Autodesk Inventor part; units mm, degrees
(part 2 of 2)
  arc A592 (44.2126, 82.716) -> (44.7772, 86.4762) centre (21.6675, 88.0234) ccw
  arc A593 (45.2915, 82.1302) -> (44.2126, 82.716) centre (0, 0) ccw
  arc A594 (48.1377, 84.6516) -> (45.2915, 82.1302) centre (62.0216, 66.1129) ccw
  arc A595 (49.2416, 84.0143) -> (48.1377, 84.6516) centre (0, 0) ccw
  arc A596 (48.481, 80.2887) -> (49.2416, 84.0143) centre (26.2446, 86.7687) ccw
  arc A597 (49.5278, 79.6472) -> (48.481, 80.2887) centre (0, 0) ccw
  arc A598 (52.502, 82.0163) -> (49.5278, 79.6472) centre (65.3967, 62.7763) ccw
  arc A599 (53.5711, 81.322) -> (52.502, 82.0163) centre (0, 0) ccw
  arc A600 (52.6166, 77.6414) -> (53.5711, 81.322) centre (30.7498, 85.2763) ccw
  arc A601 (53.6284, 76.946) -> (52.6166, 77.6414) centre (0, 0) ccw
  arc A602 (56.7225, 79.1561) -> (53.6284, 76.946) centre (68.5925, 59.2677) ccw
  arc A603 (57.7538, 78.4069) -> (56.7225, 79.1561) centre (0, 0) ccw
  arc A604 (56.6079, 74.7812) -> (57.7538, 78.4069) centre (35.1706, 83.5501) ccw
  arc A605 (57.5819, 74.0339) -> (56.6079, 74.7812) centre (0, 0) ccw
  arc A606 (60.7875, 76.079) -> (57.5819, 74.0339) centre (71.6004, 55.5966) ccw
  arc A607 (61.7781, 75.2768) -> (60.7875, 76.079) centre (0, 0) ccw
  arc A608 (60.4441, 71.7161) -> (61.7781, 75.2768) centre (39.4951, 81.5949) ccw
  arc A609 (61.3776, 70.9188) -> (60.4441, 71.7161) centre (0, 0) ccw
  arc A610 (64.6858, 72.7934) -> (61.3776, 70.9188) centre (74.4119, 51.7731) ccw
  arc A611 (65.6331, 71.9405) -> (64.6858, 72.7934) centre (0, 0) ccw
  arc A612 (64.1146, 68.4544) -> (65.6331, 71.9405) centre (43.7113, 79.4161) ccw
  arc A613 (65.0051, 67.6093) -> (64.1146, 68.4544) centre (0, 0) ccw
  arc A614 (68.4069, 69.3082) -> (65.0051, 67.6093) centre (77.0195, 47.8077) ccw
  arc A615 (69.3082, 68.4069) -> (68.4069, 69.3082) centre (0, 0) ccw
  arc A616 (67.6093, 65.0051) -> (69.3082, 68.4069) centre (47.8077, 77.0195) ccw
  arc A617 (68.4544, 64.1146) -> (67.6093, 65.0051) centre (0, 0) ccw
  arc A618 (71.9405, 65.6331) -> (68.4544, 64.1146) centre (79.4161, 43.7113) ccw
  arc A619 (72.7934, 64.6858) -> (71.9405, 65.6331) centre (0, 0) ccw
  arc A620 (70.9188, 61.3776) -> (72.7934, 64.6858) centre (51.7731, 74.4119) ccw
  arc A621 (71.7161, 60.4441) -> (70.9188, 61.3776) centre (0, 0) ccw
  arc A622 (75.2768, 61.7781) -> (71.7161, 60.4441) centre (81.5949, 39.4951) ccw
  arc A623 (76.079, 60.7875) -> (75.2768, 61.7781) centre (0, 0) ccw
  arc A624 (74.0339, 57.5819) -> (76.079, 60.7875) centre (55.5966, 71.6004) ccw
  arc A625 (74.7812, 56.6079) -> (74.0339, 57.5819) centre (0, 0) ccw
  arc A626 (78.4069, 57.7538) -> (74.7812, 56.6079) centre (83.5501, 35.1706) ccw
  arc A627 (79.1561, 56.7225) -> (78.4069, 57.7538) centre (0, 0) ccw
  arc A628 (76.946, 53.6284) -> (79.1561, 56.7225) centre (59.2677, 68.5925) ccw
  arc A629 (77.6414, 52.6166) -> (76.946, 53.6284) centre (0, 0) ccw
  arc A630 (81.322, 53.5711) -> (77.6414, 52.6166) centre (85.2763, 30.7498) ccw
  arc A631 (82.0163, 52.502) -> (81.322, 53.5711) centre (0, 0) ccw
  arc A632 (79.6472, 49.5278) -> (82.0163, 52.502) centre (62.7763, 65.3967) ccw
  arc A633 (80.2887, 48.481) -> (79.6472, 49.5278) centre (0, 0) ccw
  arc A634 (84.0143, 49.2416) -> (80.2887, 48.481) centre (86.7687, 26.2446) ccw
  arc A635 (84.6516, 48.1377) -> (84.0143, 49.2416) centre (0, 0) ccw
  arc A636 (82.1302, 45.2915) -> (84.6516, 48.1377) centre (66.1129, 62.0216) ccw
  arc A637 (82.716, 44.2126) -> (82.1302, 45.2915) centre (0, 0) ccw
  arc A638 (86.4762, 44.7772) -> (82.716, 44.2126) centre (88.0234, 21.6675) ccw
  arc A639 (87.055, 43.6414) -> (86.4762, 44.7772) centre (0, 0) ccw
  arc A640 (84.388, 40.9311) -> (87.055, 43.6414) centre (69.2682, 58.4765) ccw
  arc A641 (84.9165, 39.823) -> (84.388, 40.9311) centre (0, 0) ccw
  arc A642 (88.7012, 40.19) -> (84.9165, 39.823) centre (89.0367, 17.031) ccw
  arc A643 (89.2197, 39.0255) -> (88.7012, 40.19) centre (0, 0) ccw
  arc A644 (86.4145, 36.4585) -> (89.2197, 39.0255) centre (72.2337, 54.7712) ccw
  arc A645 (86.8843, 35.3242) -> (86.4145, 36.4585) centre (0, 0) ccw
  arc A646 (90.683, 35.4926) -> (86.8843, 35.3242) centre (89.806, 12.3479) ccw
  arc A647 (91.1398, 34.3026) -> (90.683, 35.4926) centre (0, 0) ccw
  arc A648 (88.2042, 31.8859) -> (91.1398, 34.3026) centre (75.0012, 50.9157) ccw
  arc A649 (88.614, 30.7287) -> (88.2042, 31.8859) centre (0, 0) ccw
  arc A650 (92.4163, 30.698) -> (88.614, 30.7287) centre (90.3292, 7.6309) ccw
  arc A651 (92.8102, 29.4857) -> (92.4163, 30.698) centre (0, 0) ccw
  arc A652 (89.7521, 27.226) -> (92.8102, 29.4857) centre (77.5632, 46.9207) ccw
  arc A653 (90.1008, 26.0488) -> (89.7521, 27.226) centre (0, 0) ccw
  arc A654 (93.8962, 25.8193) -> (90.1008, 26.0488) centre (90.6048, 2.8929) ccw
  arc A655 (94.2261, 24.588) -> (93.8962, 25.8193) centre (0, 0) ccw
  arc A656 (91.054, 22.4914) -> (94.2261, 24.588) centre (79.9125, 42.797) ccw
  arc A657 (91.3406, 21.2976) -> (91.054, 22.4914) centre (0, 0) ccw
  arc A658 (95.1188, 20.8697) -> (91.3406, 21.2976) centre (90.632, -1.8529) ccw
  arc A659 (95.3839, 19.6229) -> (95.1188, 20.8697) centre (0, 0) ccw
  arc A660 (92.1063, 17.6952) -> (95.3839, 19.6229) centre (82.0428, 38.5561) ccw
  arc A661 (92.33, 16.4881) -> (92.1063, 17.6952) centre (0, 0) ccw
  arc A662 (96.0807, 15.863) -> (92.33, 16.4881) centre (90.4108, -6.5937) ccw
  arc A663 (96.2801, 14.604) -> (96.0807, 15.863) centre (0, 0) ccw
  arc A664 (92.9062, 12.8505) -> (96.2801, 14.604) centre (83.9482, 34.2094) ccw
  arc A665 (93.0664, 11.6333) -> (92.9062, 12.8505) centre (0, 0) ccw
  arc A666 (96.7792, 10.8128) -> (93.0664, 11.6333) centre (89.9418, -11.3164) ccw
  arc A667 (96.9125, 9.545) -> (96.7792, 10.8128) centre (0, 0) ccw
  arc A668 (93.4514, 7.9705) -> (96.9125, 9.545) centre (85.6236, 29.769) ccw
  arc A669 (93.5477, 6.7466) -> (93.4514, 7.9705) centre (0, 0) ccw
  arc A670 (97.2125, 5.7329) -> (93.5477, 6.7466) centre (89.2263, -16.0081) ccw
  arc A671 (97.2792, 4.46) -> (97.2125, 5.7329) centre (0, 0) ccw
  arc A672 (93.7404, 3.0687) -> (97.2792, 4.46) centre (87.0642, 25.2471) ccw
  arc A673 (93.7726, 1.8415) -> (93.7404, 3.0687) centre (0, 0) ccw
  arc A674 (97.3793, 0.6374) -> (93.7726, 1.8415) centre (88.2662, -20.6559) ccw
  arc A675 (97.3793, -0.6374) -> (97.3793, 0.6374) centre (0, 0) ccw
  arc A676 (93.7726, -1.8415) -> (97.3793, -0.6374) centre (88.2662, 20.6559) ccw
  arc A677 (93.7404, -3.0687) -> (93.7726, -1.8415) centre (0, 0) ccw
  arc A678 (97.2792, -4.46) -> (93.7404, -3.0687) centre (87.0642, -25.2471) ccw
  arc A679 (97.2125, -5.7329) -> (97.2792, -4.46) centre (0, 0) ccw
  arc A680 (93.5477, -6.7466) -> (97.2125, -5.7329) centre (89.2263, 16.0081) ccw
  arc A681 (93.4514, -7.9705) -> (93.5477, -6.7466) centre (0, 0) ccw
  arc A682 (96.9125, -9.545) -> (93.4514, -7.9705) centre (85.6236, -29.769) ccw
  arc A683 (96.7792, -10.8128) -> (96.9125, -9.545) centre (0, 0) ccw
  arc A684 (93.0664, -11.6333) -> (96.7792, -10.8128) centre (89.9418, 11.3164) ccw
  arc A685 (92.9062, -12.8505) -> (93.0664, -11.6333) centre (0, 0) ccw
  arc A686 (96.2801, -14.604) -> (92.9062, -12.8505) centre (83.9482, -34.2094) ccw
  arc A687 (96.0807, -15.863) -> (96.2801, -14.604) centre (0, 0) ccw
  arc A688 (92.33, -16.4881) -> (96.0807, -15.863) centre (90.4108, 6.5937) ccw
  arc A689 (92.1063, -17.6952) -> (92.33, -16.4881) centre (0, 0) ccw
  arc A690 (95.3839, -19.6229) -> (92.1063, -17.6952) centre (82.0428, -38.5561) ccw
  arc A691 (95.1188, -20.8697) -> (95.3839, -19.6229) centre (0, 0) ccw
  arc A692 (91.3406, -21.2976) -> (95.1188, -20.8697) centre (90.632, 1.8529) ccw
  arc A693 (91.054, -22.4914) -> (91.3406, -21.2976) centre (0, 0) ccw
  arc A694 (94.2261, -24.588) -> (91.054, -22.4914) centre (79.9125, -42.797) ccw
  arc A695 (93.8962, -25.8193) -> (94.2261, -24.588) centre (0, 0) ccw
  arc A696 (90.1008, -26.0488) -> (93.8962, -25.8193) centre (90.6048, -2.8929) ccw
  arc A697 (89.7521, -27.226) -> (90.1008, -26.0488) centre (0, 0) ccw
  arc A698 (92.8102, -29.4857) -> (89.7521, -27.226) centre (77.5632, -46.9207) ccw
  arc A699 (92.4163, -30.698) -> (92.8102, -29.4857) centre (0, 0) ccw
  arc A700 (88.614, -30.7287) -> (92.4163, -30.698) centre (90.3292, -7.6309) ccw
  arc A701 (88.2042, -31.8859) -> (88.614, -30.7287) centre (0, 0) ccw
  arc A702 (91.1398, -34.3026) -> (88.2042, -31.8859) centre (75.0012, -50.9157) ccw
  arc A703 (90.683, -35.4926) -> (91.1398, -34.3026) centre (0, 0) ccw
  arc A704 (86.8843, -35.3242) -> (90.683, -35.4926) centre (89.806, -12.3479) ccw
  arc A705 (86.4145, -36.4585) -> (86.8843, -35.3242) centre (0, 0) ccw
  arc A706 (89.2197, -39.0255) -> (86.4145, -36.4585) centre (72.2337, -54.7712) ccw
  arc A707 (88.7012, -40.19) -> (89.2197, -39.0255) centre (0, 0) ccw
  arc A708 (84.9165, -39.823) -> (88.7012, -40.19) centre (89.0367, -17.031) ccw
  arc A709 (84.388, -40.9311) -> (84.9165, -39.823) centre (0, 0) ccw
  arc A710 (87.055, -43.6414) -> (84.388, -40.9311) centre (69.2682, -58.4765) ccw
  arc A711 (86.4762, -44.7772) -> (87.055, -43.6414) centre (0, 0) ccw
  arc A712 (82.716, -44.2126) -> (86.4762, -44.7772) centre (88.0234, -21.6675) ccw
  arc A713 (82.1302, -45.2915) -> (82.716, -44.2126) centre (0, 0) ccw
  arc A714 (84.6516, -48.1377) -> (82.1302, -45.2915) centre (66.1129, -62.0216) ccw
  arc A715 (84.0143, -49.2416) -> (84.6516, -48.1377) centre (0, 0) ccw
  arc A716 (80.2887, -48.481) -> (84.0143, -49.2416) centre (86.7687, -26.2446) ccw
  arc A717 (79.6472, -49.5278) -> (80.2887, -48.481) centre (0, 0) ccw
  arc A718 (82.0163, -52.502) -> (79.6472, -49.5278) centre (62.7763, -65.3967) ccw
  arc A719 (81.322, -53.5711) -> (82.0163, -52.502) centre (0, 0) ccw
  arc A720 (77.6414, -52.6166) -> (81.322, -53.5711) centre (85.2763, -30.7498) ccw
  arc A721 (76.946, -53.6284) -> (77.6414, -52.6166) centre (0, 0) ccw
  arc A722 (79.1561, -56.7225) -> (76.946, -53.6284) centre (59.2677, -68.5925) ccw
  arc A723 (78.4069, -57.7538) -> (79.1561, -56.7225) centre (0, 0) ccw
  arc A724 (74.7812, -56.6079) -> (78.4069, -57.7538) centre (83.5501, -35.1706) ccw
  arc A725 (74.0339, -57.5819) -> (74.7812, -56.6079) centre (0, 0) ccw
  arc A726 (76.079, -60.7875) -> (74.0339, -57.5819) centre (55.5966, -71.6004) ccw
  arc A727 (75.2768, -61.7781) -> (76.079, -60.7875) centre (0, 0) ccw
  arc A728 (71.7161, -60.4441) -> (75.2768, -61.7781) centre (81.5949, -39.4951) ccw
  arc A729 (70.9188, -61.3776) -> (71.7161, -60.4441) centre (0, 0) ccw
  arc A730 (72.7934, -64.6858) -> (70.9188, -61.3776) centre (51.7731, -74.4119) ccw
  arc A731 (71.9405, -65.6331) -> (72.7934, -64.6858) centre (0, 0) ccw
  arc A732 (68.4544, -64.1146) -> (71.9405, -65.6331) centre (79.4161, -43.7113) ccw
  arc A733 (67.6093, -65.0051) -> (68.4544, -64.1146) centre (0, 0) ccw
  arc A734 (69.3082, -68.4069) -> (67.6093, -65.0051) centre (47.8077, -77.0195) ccw
  arc A735 (68.4069, -69.3082) -> (69.3082, -68.4069) centre (0, 0) ccw
  arc A736 (65.0051, -67.6093) -> (68.4069, -69.3082) centre (77.0195, -47.8077) ccw
  arc A737 (64.1146, -68.4544) -> (65.0051, -67.6093) centre (0, 0) ccw
  arc A738 (65.6331, -71.9405) -> (64.1146, -68.4544) centre (43.7113, -79.4161) ccw
  arc A739 (64.6858, -72.7934) -> (65.6331, -71.9405) centre (0, 0) ccw
  arc A740 (61.3776, -70.9188) -> (64.6858, -72.7934) centre (74.4119, -51.7731) ccw
  arc A741 (60.4441, -71.7161) -> (61.3776, -70.9188) centre (0, 0) ccw
  arc A742 (61.7781, -75.2768) -> (60.4441, -71.7161) centre (39.4951, -81.5949) ccw
  arc A743 (60.7875, -76.079) -> (61.7781, -75.2768) centre (0, 0) ccw
  arc A744 (57.5819, -74.0339) -> (60.7875, -76.079) centre (71.6004, -55.5966) ccw
  arc A745 (56.6079, -74.7812) -> (57.5819, -74.0339) centre (0, 0) ccw
  arc A746 (57.7538, -78.4069) -> (56.6079, -74.7812) centre (35.1706, -83.5501) ccw
  arc A747 (56.7225, -79.1561) -> (57.7538, -78.4069) centre (0, 0) ccw
  arc A748 (53.6284, -76.946) -> (56.7225, -79.1561) centre (68.5925, -59.2677) ccw
  arc A749 (52.6166, -77.6414) -> (53.6284, -76.946) centre (0, 0) ccw
  arc A750 (53.5711, -81.322) -> (52.6166, -77.6414) centre (30.7498, -85.2763) ccw
  arc A751 (52.502, -82.0163) -> (53.5711, -81.322) centre (0, 0) ccw
  arc A752 (49.5278, -79.6472) -> (52.502, -82.0163) centre (65.3967, -62.7763) ccw
  arc A753 (48.481, -80.2887) -> (49.5278, -79.6472) centre (0, 0) ccw
  arc A754 (49.2416, -84.0143) -> (48.481, -80.2887) centre (26.2446, -86.7687) ccw
  arc A755 (48.1377, -84.6516) -> (49.2416, -84.0143) centre (0, 0) ccw
  arc A756 (45.2915, -82.1302) -> (48.1377, -84.6516) centre (62.0216, -66.1129) ccw
  arc A757 (44.2126, -82.716) -> (45.2915, -82.1302) centre (0, 0) ccw
  arc A758 (44.7772, -86.4762) -> (44.2126, -82.716) centre (21.6675, -88.0234) ccw
  arc A759 (43.6414, -87.055) -> (44.7772, -86.4762) centre (0, 0) ccw
  arc A760 (40.9311, -84.388) -> (43.6414, -87.055) centre (58.4765, -69.2682) ccw
  arc A761 (39.823, -84.9165) -> (40.9311, -84.388) centre (0, 0) ccw
  arc A762 (40.19, -88.7012) -> (39.823, -84.9165) centre (17.031, -89.0367) ccw
  arc A763 (39.0255, -89.2197) -> (40.19, -88.7012) centre (0, 0) ccw
  arc A764 (36.4585, -86.4145) -> (39.0255, -89.2197) centre (54.7712, -72.2337) ccw
  arc A765 (35.3242, -86.8843) -> (36.4585, -86.4145) centre (0, 0) ccw
  arc A766 (35.4926, -90.683) -> (35.3242, -86.8843) centre (12.3479, -89.806) ccw
  arc A767 (34.3026, -91.1398) -> (35.4926, -90.683) centre (0, 0) ccw
  arc A768 (31.8859, -88.2042) -> (34.3026, -91.1398) centre (50.9157, -75.0012) ccw
  arc A769 (30.7287, -88.614) -> (31.8859, -88.2042) centre (0, 0) ccw
  arc A770 (30.698, -92.4163) -> (30.7287, -88.614) centre (7.6309, -90.3292) ccw
  arc A771 (29.4857, -92.8102) -> (30.698, -92.4163) centre (0, 0) ccw
  arc A772 (27.226, -89.7521) -> (29.4857, -92.8102) centre (46.9207, -77.5632) ccw
  arc A773 (26.0488, -90.1008) -> (27.226, -89.7521) centre (0, 0) ccw
  arc A774 (25.8193, -93.8962) -> (26.0488, -90.1008) centre (2.8929, -90.6048) ccw
  arc A775 (24.588, -94.2261) -> (25.8193, -93.8962) centre (0, 0) ccw
  arc A776 (22.4914, -91.054) -> (24.588, -94.2261) centre (42.797, -79.9125) ccw
  arc A777 (21.2976, -91.3406) -> (22.4914, -91.054) centre (0, 0) ccw
  arc A778 (20.8697, -95.1188) -> (21.2976, -91.3406) centre (-1.8529, -90.632) ccw
  arc A779 (19.6229, -95.3839) -> (20.8697, -95.1188) centre (0, 0) ccw
  arc A780 (17.6952, -92.1063) -> (19.6229, -95.3839) centre (38.5561, -82.0428) ccw
  arc A781 (16.4881, -92.33) -> (17.6952, -92.1063) centre (0, 0) ccw
  arc A782 (15.863, -96.0807) -> (16.4881, -92.33) centre (-6.5937, -90.4108) ccw
  arc A783 (14.604, -96.2801) -> (15.863, -96.0807) centre (0, 0) ccw
  arc A784 (12.8505, -92.9062) -> (14.604, -96.2801) centre (34.2094, -83.9482) ccw
  arc A785 (11.6333, -93.0664) -> (12.8505, -92.9062) centre (0, 0) ccw
  arc A786 (10.8128, -96.7792) -> (11.6333, -93.0664) centre (-11.3164, -89.9418) ccw
  arc A787 (9.545, -96.9125) -> (10.8128, -96.7792) centre (0, 0) ccw
  arc A788 (7.9705, -93.4514) -> (9.545, -96.9125) centre (29.769, -85.6236) ccw
  arc A789 (6.7466, -93.5477) -> (7.9705, -93.4514) centre (0, 0) ccw
  arc A790 (5.7329, -97.2125) -> (6.7466, -93.5477) centre (-16.0081, -89.2263) ccw
  arc A791 (4.46, -97.2792) -> (5.7329, -97.2125) centre (0, 0) ccw
  arc A792 (3.0687, -93.7404) -> (4.46, -97.2792) centre (25.2471, -87.0642) ccw
  arc A793 (1.8415, -93.7726) -> (3.0687, -93.7404) centre (0, 0) ccw
  arc A794 (0.6374, -97.3793) -> (1.8415, -93.7726) centre (-20.6559, -88.2662) ccw
  arc A795 (-0.6374, -97.3793) -> (0.6374, -97.3793) centre (0, 0) ccw
  arc A796 (-1.8415, -93.7726) -> (-0.6374, -97.3793) centre (20.6559, -88.2662) ccw
  arc A797 (-3.0687, -93.7404) -> (-1.8415, -93.7726) centre (0, 0) ccw
  arc A798 (-4.46, -97.2792) -> (-3.0687, -93.7404) centre (-25.2471, -87.0642) ccw
  arc A799 (-5.7329, -97.2125) -> (-4.46, -97.2792) centre (0, 0) ccw
  circle A800 centre (0, 0) radius 107.1195
  point P0 (-22.0768, -1.1949)
  point P1 (-22.0768, 62.1365)
  point P2 (11.0298, -31.6657)
  point P3 (-11.0298, -31.6657)
  point P4 (-9.3264, -31.6657)
  point P5 (-6.2126, -31.6657)
  point P6 (-3.6909, -31.6657)
  point P7 (-1.3643, -31.6657)
  point P8 (1.3643, -31.6657)
  point P9 (3.6909, -31.6657)
  point P10 (6.2126, -31.6657)
  point P11 (9.3264, -31.6657)
  constraints: 1600 point on circle, 801 centre point
extrude "Extrusion2" add sketch "Sketch3" against normal blind 3 contours A800
sketch "Sketch4" plane through (0, 0, 0) normal (1, 0, 0) x (0, 0, -1)
  line L0 (-178, 76) -> (151, 76)
  line L1 (151, 76) -> (151, -19)
  line L2 (151, -19) -> (-178, -19)
  line L3 (-178, -19) -> (-178, 76)
  point P0 (0, 0)
  constraints: 8 end point, 2 parallel, 1 horizontal, 1 perpendicular
extrude "Extrusion3" cut sketch "Sketch4" along normal blind 136
sketch "Sketch5" plane through (0, 0, 0) normal (0, 0, 1) x (1, 0, 0)
  line L0 (29, 45) -> (-152, 45)
  line L1 (-152, 45) -> (-152, -11)
  line L2 (-152, -11) -> (29, -11)
  line L3 (29, -11) -> (29, 45)
  point P0 (0, 0)
  constraints: 8 end point, 2 parallel, 1 horizontal, 1 perpendicular
extrude "Extrusion4" cut sketch "Sketch5" against normal blind 174
fillet "Fillet2" radius 2 1 edges at (-72.9985, 11.9, 72.9985)
sketch "Sketch6" plane through (0, 8.9, 97.3814) normal (0, -1, 0) x (1, 0, 0)
  line L0 (-113.2355, -97.3814) -> (-97.3814, -97.3814) projected
  arc A0 (-97.3793, -96.744) -> (-97.3814, -97.3814) centre (0, -97.3814) ccw projected
  arc A1 (-93.7726, -95.5399) -> (-97.3793, -96.744) centre (-88.2662, -118.0373) ccw projected
  arc A2 (-93.7404, -94.3127) -> (-93.7726, -95.5399) centre (0, -97.3814) ccw projected
  arc A3 (-97.2792, -92.9214) -> (-93.7404, -94.3127) centre (-87.0642, -72.1343) ccw projected
  arc A4 (-97.2125, -91.6485) -> (-97.2792, -92.9214) centre (0, -97.3814) ccw projected
  arc A5 (-93.5477, -90.6348) -> (-97.2125, -91.6485) centre (-89.2263, -113.3895) ccw projected
  arc A6 (-93.4514, -89.4109) -> (-93.5477, -90.6348) centre (0, -97.3814) ccw projected
  arc A7 (-96.9125, -87.8363) -> (-93.4514, -89.4109) centre (-85.6236, -67.6124) ccw projected
  arc A8 (-96.7792, -86.5686) -> (-96.9125, -87.8363) centre (0, -97.3814) ccw projected
  arc A9 (-93.0664, -85.7481) -> (-96.7792, -86.5686) centre (-89.9418, -108.6978) ccw projected
  arc A10 (-92.9062, -84.5309) -> (-93.0664, -85.7481) centre (0, -97.3814) ccw projected
  arc A11 (-96.2801, -82.7774) -> (-92.9062, -84.5309) centre (-83.9482, -63.172) ccw projected
  arc A12 (-96.0807, -81.5184) -> (-96.2801, -82.7774) centre (0, -97.3814) ccw projected
  arc A13 (-92.33, -80.8933) -> (-96.0807, -81.5184) centre (-90.4108, -103.9751) ccw projected
  arc A14 (-92.1063, -79.6862) -> (-92.33, -80.8933) centre (0, -97.3814) ccw projected
  arc A15 (-95.3839, -77.7585) -> (-92.1063, -79.6862) centre (-82.0428, -58.8253) ccw projected
  arc A16 (-95.1188, -76.5117) -> (-95.3839, -77.7585) centre (0, -97.3814) ccw projected
  arc A17 (-91.3406, -76.0838) -> (-95.1188, -76.5117) centre (-90.632, -99.2343) ccw projected
  arc A18 (-91.054, -74.89) -> (-91.3406, -76.0838) centre (0, -97.3814) ccw projected
  arc A19 (-94.2261, -72.7934) -> (-91.054, -74.89) centre (-79.9125, -54.5844) ccw projected
  arc A20 (-93.8962, -71.5621) -> (-94.2261, -72.7934) centre (0, -97.3814) ccw projected
  arc A21 (-90.1008, -71.3326) -> (-93.8962, -71.5621) centre (-90.6048, -94.4884) ccw projected
  arc A22 (-89.7521, -70.1554) -> (-90.1008, -71.3326) centre (0, -97.3814) ccw projected
  arc A23 (-92.8102, -67.8957) -> (-89.7521, -70.1554) centre (-77.5632, -50.4607) ccw projected
  arc A24 (-92.4163, -66.6834) -> (-92.8102, -67.8957) centre (0, -97.3814) ccw projected
  arc A25 (-88.614, -66.6527) -> (-92.4163, -66.6834) centre (-90.3292, -89.7505) ccw projected
  arc A26 (-88.2042, -65.4955) -> (-88.614, -66.6527) centre (0, -97.3814) ccw projected
  arc A27 (-91.1398, -63.0788) -> (-88.2042, -65.4955) centre (-75.0012, -46.4657) ccw projected
  arc A28 (-90.683, -61.8887) -> (-91.1398, -63.0788) centre (0, -97.3814) ccw projected
  arc A29 (-86.8843, -62.0572) -> (-90.683, -61.8887) centre (-89.806, -85.0335) ccw projected
  arc A30 (-86.4145, -60.9229) -> (-86.8843, -62.0572) centre (0, -97.3814) ccw projected
  arc A31 (-89.2197, -58.3559) -> (-86.4145, -60.9229) centre (-72.2337, -42.6102) ccw projected
  arc A32 (-88.7012, -57.1914) -> (-89.2197, -58.3559) centre (0, -97.3814) ccw projected
  arc A33 (-84.9165, -57.5584) -> (-88.7012, -57.1914) centre (-89.0367, -80.3504) ccw projected
  arc A34 (-84.388, -56.4503) -> (-84.9165, -57.5584) centre (0, -97.3814) ccw projected
  arc A35 (-87.055, -53.74) -> (-84.388, -56.4503) centre (-69.2682, -38.9049) ccw projected
  arc A36 (-86.4762, -52.6042) -> (-87.055, -53.74) centre (0, -97.3814) ccw projected
  arc A37 (-82.716, -53.1688) -> (-86.4762, -52.6042) centre (-88.0234, -75.7139) ccw projected
  arc A38 (-82.1302, -52.0899) -> (-82.716, -53.1688) centre (0, -97.3814) ccw projected
  arc A39 (-84.6516, -49.2437) -> (-82.1302, -52.0899) centre (-66.1129, -35.3598) ccw projected
  arc A40 (-84.0143, -48.1398) -> (-84.6516, -49.2437) centre (0, -97.3814) ccw projected
  arc A41 (-80.2887, -48.9004) -> (-84.0143, -48.1398) centre (-86.7687, -71.1368) ccw projected
  arc A42 (-79.6472, -47.8536) -> (-80.2887, -48.9004) centre (0, -97.3814) ccw projected
  arc A43 (-82.0163, -44.8794) -> (-79.6472, -47.8536) centre (-62.7763, -31.9847) ccw projected
  arc A44 (-81.322, -43.8103) -> (-82.0163, -44.8794) centre (0, -97.3814) ccw projected
  arc A45 (-77.6414, -44.7648) -> (-81.322, -43.8103) centre (-85.2763, -66.6316) ccw projected
  arc A46 (-76.946, -43.753) -> (-77.6414, -44.7648) centre (0, -97.3814) ccw projected
  arc A47 (-79.1561, -40.6589) -> (-76.946, -43.753) centre (-59.2677, -28.7889) ccw projected
  arc A48 (-78.4069, -39.6276) -> (-79.1561, -40.6589) centre (0, -97.3814) ccw projected
  arc A49 (-74.7812, -40.7735) -> (-78.4069, -39.6276) centre (-83.5501, -62.2108) ccw projected
  arc A50 (-74.0339, -39.7995) -> (-74.7812, -40.7735) centre (0, -97.3814) ccw projected
  arc A51 (-76.079, -36.5939) -> (-74.0339, -39.7995) centre (-55.5966, -25.781) ccw projected
  arc A52 (-75.2768, -35.6033) -> (-76.079, -36.5939) centre (0, -97.3814) ccw projected
  arc A53 (-71.7161, -36.9373) -> (-75.2768, -35.6033) centre (-81.5949, -57.8863) ccw projected
  arc A54 (-70.9188, -36.0038) -> (-71.7161, -36.9373) centre (0, -97.3814) ccw projected
  arc A55 (-72.7934, -32.6956) -> (-70.9188, -36.0038) centre (-51.7731, -22.9695) ccw projected
  arc A56 (-71.9405, -31.7483) -> (-72.7934, -32.6956) centre (0, -97.3814) ccw projected
  arc A57 (-68.4544, -33.2668) -> (-71.9405, -31.7483) centre (-79.4161, -53.6701) ccw projected
  arc A58 (-67.6093, -32.3763) -> (-68.4544, -33.2668) centre (0, -97.3814) ccw projected
  arc A59 (-69.3082, -28.9745) -> (-67.6093, -32.3763) centre (-47.8077, -20.3618) ccw projected
  arc A60 (-68.4069, -28.0731) -> (-69.3082, -28.9745) centre (0, -97.3814) ccw projected
  arc A61 (-65.0051, -29.7721) -> (-68.4069, -28.0731) centre (-77.0195, -49.5736) ccw projected
  arc A62 (-64.1146, -28.927) -> (-65.0051, -29.7721) centre (0, -97.3814) ccw projected
  arc A63 (-65.6331, -25.4409) -> (-64.1146, -28.927) centre (-43.7113, -17.9653) ccw projected
  arc A64 (-64.6858, -24.588) -> (-65.6331, -25.4409) centre (0, -97.3814) ccw projected
  arc A65 (-61.3776, -26.4626) -> (-64.6858, -24.588) centre (-74.4119, -45.6083) ccw projected
  arc A66 (-60.4441, -25.6653) -> (-61.3776, -26.4626) centre (0, -97.3814) ccw projected
  arc A67 (-61.7781, -22.1046) -> (-60.4441, -25.6653) centre (-39.4951, -15.7865) ccw projected
  arc A68 (-60.7875, -21.3024) -> (-61.7781, -22.1046) centre (0, -97.3814) ccw projected
  arc A69 (-57.5819, -23.3475) -> (-60.7875, -21.3024) centre (-71.6004, -41.7848) ccw projected
  arc A70 (-56.6079, -22.6002) -> (-57.5819, -23.3475) centre (0, -97.3814) ccw projected
  arc A71 (-57.7538, -18.9745) -> (-56.6079, -22.6002) centre (-35.1706, -13.8313) ccw projected
  arc A72 (-56.7225, -18.2253) -> (-57.7538, -18.9745) centre (0, -97.3814) ccw projected
  arc A73 (-53.6284, -20.4354) -> (-56.7225, -18.2253) centre (-68.5925, -38.1137) ccw projected
  arc A74 (-52.6166, -19.74) -> (-53.6284, -20.4354) centre (0, -97.3814) ccw projected
  arc A75 (-53.5711, -16.0594) -> (-52.6166, -19.74) centre (-30.7498, -12.1051) ccw projected
  arc A76 (-52.502, -15.3651) -> (-53.5711, -16.0594) centre (0, -97.3814) ccw projected
  arc A77 (-49.5278, -17.7342) -> (-52.502, -15.3651) centre (-65.3967, -34.6051) ccw projected
  arc A78 (-48.481, -17.0927) -> (-49.5278, -17.7342) centre (0, -97.3814) ccw projected
  arc A79 (-49.2416, -13.3671) -> (-48.481, -17.0927) centre (-26.2446, -10.6127) ccw projected
  arc A80 (-48.1377, -12.7298) -> (-49.2416, -13.3671) centre (0, -97.3814) ccw projected
  arc A81 (-45.2915, -15.2512) -> (-48.1377, -12.7298) centre (-62.0216, -31.2685) ccw projected
  arc A82 (-44.2126, -14.6654) -> (-45.2915, -15.2512) centre (0, -97.3814) ccw projected
  arc A83 (-44.7772, -10.9051) -> (-44.2126, -14.6654) centre (-21.6675, -9.358) ccw projected
  arc A84 (-43.6414, -10.3264) -> (-44.7772, -10.9051) centre (0, -97.3814) ccw projected
  arc A85 (-40.9311, -12.9934) -> (-43.6414, -10.3264) centre (-58.4765, -28.1132) ccw projected
  arc A86 (-39.823, -12.4649) -> (-40.9311, -12.9934) centre (0, -97.3814) ccw projected
  arc A87 (-40.19, -8.6802) -> (-39.823, -12.4649) centre (-17.031, -8.3447) ccw projected
  arc A88 (-39.0255, -8.1617) -> (-40.19, -8.6802) centre (0, -97.3814) ccw projected
  arc A89 (-36.4585, -10.9669) -> (-39.0255, -8.1617) centre (-54.7712, -25.1477) ccw projected
  arc A90 (-35.3242, -10.4971) -> (-36.4585, -10.9669) centre (0, -97.3814) ccw projected
  arc A91 (-35.4926, -6.6984) -> (-35.3242, -10.4971) centre (-12.3479, -7.5754) ccw projected
  arc A92 (-34.3026, -6.2416) -> (-35.4926, -6.6984) centre (0, -97.3814) ccw projected
  arc A93 (-31.8859, -9.1772) -> (-34.3026, -6.2416) centre (-50.9157, -22.3802) ccw projected
  arc A94 (-30.7287, -8.7674) -> (-31.8859, -9.1772) centre (0, -97.3814) ccw projected
  arc A95 (-30.698, -4.9651) -> (-30.7287, -8.7674) centre (-7.6309, -7.0522) ccw projected
  arc A96 (-29.4857, -4.5712) -> (-30.698, -4.9651) centre (0, -97.3814) ccw projected
  arc A97 (-27.226, -7.6293) -> (-29.4857, -4.5712) centre (-46.9207, -19.8182) ccw projected
  arc A98 (-26.0488, -7.2806) -> (-27.226, -7.6293) centre (0, -97.3814) ccw projected
  arc A99 (-25.8193, -3.4852) -> (-26.0488, -7.2806) centre (-2.8929, -6.7766) ccw projected
  arc A100 (-24.588, -3.1552) -> (-25.8193, -3.4852) centre (0, -97.3814) ccw projected
  arc A101 (-22.4914, -6.3274) -> (-24.588, -3.1552) centre (-42.797, -17.4689) ccw projected
  arc A102 (-21.2976, -6.0408) -> (-22.4914, -6.3274) centre (0, -97.3814) ccw projected
  arc A103 (-20.8697, -2.2626) -> (-21.2976, -6.0408) centre (1.8529, -6.7494) ccw projected
  arc A104 (-19.6229, -1.9975) -> (-20.8697, -2.2626) centre (0, -97.3814) ccw projected
  arc A105 (-17.6952, -5.2751) -> (-19.6229, -1.9975) centre (-38.5561, -15.3386) ccw projected
  arc A106 (-16.4881, -5.0514) -> (-17.6952, -5.2751) centre (0, -97.3814) ccw projected
  arc A107 (-15.863, -1.3007) -> (-16.4881, -5.0514) centre (6.5937, -6.9706) ccw projected
  arc A108 (-14.604, -1.1013) -> (-15.863, -1.3007) centre (0, -97.3814) ccw projected
  arc A109 (-12.8505, -4.4752) -> (-14.604, -1.1013) centre (-34.2094, -13.4332) ccw projected
  arc A110 (-11.6333, -4.315) -> (-12.8505, -4.4752) centre (0, -97.3814) ccw projected
  arc A111 (-10.8128, -0.6022) -> (-11.6333, -4.315) centre (11.3164, -7.4396) ccw projected
  arc A112 (-9.545, -0.4689) -> (-10.8128, -0.6022) centre (0, -97.3814) ccw projected
  arc A113 (-7.9705, -3.93) -> (-9.545, -0.4689) centre (-29.769, -11.7578) ccw projected
  arc A114 (-6.7466, -3.8337) -> (-7.9705, -3.93) centre (0, -97.3814) ccw projected
  arc A115 (-5.7329, -0.1689) -> (-6.7466, -3.8337) centre (16.0081, -8.1551) ccw projected
  arc A116 (-4.46, -0.1022) -> (-5.7329, -0.1689) centre (0, -97.3814) ccw projected
  arc A117 (-3.0687, -3.6409) -> (-4.46, -0.1022) centre (-25.2471, -10.3172) ccw projected
  arc A118 (-1.8415, -3.6088) -> (-3.0687, -3.6409) centre (0, -97.3814) ccw projected
  arc A119 (-0.6374, -0.0021) -> (-1.8415, -3.6088) centre (20.6559, -9.1152) ccw projected
  arc A120 (0, 0) -> (-0.6374, -0.0021) centre (0, -97.3814) ccw projected
  line L1 (0, 0) -> (0, 15.8541) projected
  arc A121 (0, 15.8541) -> (-113.2355, -97.3814) centre (0, -97.3814) ccw projected
  line L2 (0, 0) -> (0, 15.8541) projected
  line L3 (0, 7.9271) -> (0, 10.4271)
  line L4 (0, 10.4271) -> (0, 12.4271)
  line L5 (0, 12.4271) -> (-5, 12.4271)
  line L6 (-5, 12.4271) -> (-5, 14.9271)
  line L7 (-5, 14.9271) -> (-10, 14.9271)
  line L8 (-10, 14.9271) -> (-10, 4.9271)
  line L9 (-10, 4.9271) -> (-5, 4.9271)
  line L10 (-5, 4.9271) -> (-5, 7.4271)
  line L11 (-5, 7.4271) -> (0, 7.4271)
  line L12 (0, -97.3814) -> (-115.3814, 18)
  line L13 (0, -97.3814) -> (163.1739, -97.3814) construction
  line L14 (-109.8085, -92.3814) -> (-112.3085, -92.3814)
  line L15 (-102.3085, -87.3814) -> (-102.3085, -92.3814)
  line L16 (-112.3085, -87.3814) -> (-102.3085, -87.3814)
  line L17 (-112.3085, -92.3814) -> (-112.3085, -87.3814)
  line L18 (-109.8085, -97.3814) -> (-109.8085, -92.3814)
  line L19 (-102.3085, -92.3814) -> (-104.8085, -92.3814)
  line L20 (-104.8085, -92.3814) -> (-104.8085, -97.3814)
  point P0 (0, 7.4271)
  point P1 (0, 12.4271)
  dimension "d17" = 2.5
  dimension "d27" = 2
  dimension "d28" = 5
  dimension "d29" = 2.5
  dimension "d30" = 90
  dimension "d31" = 5
  dimension "d32" = 10
  dimension "d33" = 5
  dimension "d34" = 2.5
  dimension "d36" = 135
  constraints: 36 end point, 8 symmetric about line, 4 perpendicular, 2 horizontal, 2 point on line, 1 equal length, 1 midpoint
  measures "d17" distance of L3.start L3.end
  measures "d27" distance of L3.end L4.end
  measures "d28" distance of L5.start L6.start
  measures "d29" distance of L6.start L6.end
  measures "d30" angle of L5 L6
  measures "d31" distance of L6.end L8.start
  measures "d32" distance of L8.start L9.start
  measures "d33" distance of L9.start L9.end
  measures "d34" distance of L9.end L10.end
  measures "d36" angle of L13 L12
extrude "Extrusion5" cut sketch "Sketch6" against normal blind 3 contours L18 L14 L17 L16 L15 L19 L20 L0 | L1 L11 L10 L9 L8 L7 L6 L5
fillet "Fillet3" radius 2 1 edges at (-72.9985, 15.9, 72.9985)
fillet "Fillet4" radius 1 4 edges at (-94.2117, 15.9, 94.2117) (-94.2117, 8.9, 94.2117) (-87.1407, 8.9, 87.1407) (-80.0696, 8.9, 80.0696)
body "Solid1"
